Autodesk Fusion 360 part; units mm, degrees
(part 5 of 5)
  line L3475 (115.1928, -67.2452) -> (117.5491, -67.2452)
  line L3476 (117.5491, -67.2452) -> (117.5491, -64.2936)
  line L3477 (117.5491, -64.2936) -> (117.551, -64.2841)
  line L3478 (117.551, -64.2841) -> (117.5645, -64.2705)
  line L3479 (117.5645, -64.2705) -> (117.5741, -64.2686)
  line L3480 (117.5741, -64.2686) -> (131.2663, -64.2686)
  line L3481 (131.2663, -64.2686) -> (131.2758, -64.2705)
  line L3482 (117.5991, -64.3186) -> (117.5991, -67.2702)
  line L3483 (117.5991, -67.2702) -> (117.5972, -67.2798)
  line L3484 (117.5972, -67.2798) -> (117.5836, -67.2933)
  line L3485 (117.5836, -67.2933) -> (117.5741, -67.2952)
  line L3486 (117.5741, -67.2952) -> (115.2178, -67.2952)
  line L3487 (115.2178, -67.2952) -> (115.2178, -70.5194)
  line L3488 (115.2178, -70.5194) -> (117.5741, -70.5194)
  line L3489 (117.5741, -70.5194) -> (117.5836, -70.5213)
  line L3490 (117.5836, -70.5213) -> (117.5972, -70.5348)
  line L3491 (117.5972, -70.5348) -> (117.5991, -70.5444)
  line L3492 (117.5991, -70.5444) -> (117.5991, -72.603)
  line L3493 (117.5991, -72.603) -> (119.9303, -72.603)
  line L3494 (119.9303, -72.603) -> (119.9303, -70.8421)
  line L3495 (119.9303, -70.8421) -> (119.9322, -70.8325)
  line L3496 (119.9322, -70.8325) -> (119.9458, -70.819)
  line L3497 (119.9458, -70.819) -> (119.9553, -70.8171)
  line L3498 (119.9553, -70.8171) -> (121.4436, -70.8171)
  line L3499 (121.4436, -70.8171) -> (121.4532, -70.819)
  line L3500 (121.4532, -70.819) -> (121.4667, -70.8325)
  line L3501 (121.4667, -70.8325) -> (121.4686, -70.8421)
  line L3502 (121.4686, -70.8421) -> (121.4686, -73.7936)
  line L3503 (121.4686, -73.7936) -> (121.7413, -73.7936)
  line L3504 (121.7413, -73.7936) -> (126.1811, -73.7936)
  line L3505 (126.1811, -73.7936) -> (126.1811, -72.628)
  line L3506 (126.1811, -72.628) -> (126.1811, -68.7585)
  line L3507 (126.1811, -68.7585) -> (126.183, -68.7489)
  line L3508 (126.183, -68.7489) -> (126.1965, -68.7354)
  line L3509 (126.1965, -68.7354) -> (126.2061, -68.7335)
  line L3510 (126.2061, -68.7335) -> (128.86, -68.7335)
  line L3511 (128.86, -68.7335) -> (128.86, -67.8655)
  line L3512 (128.86, -67.8655) -> (128.8619, -67.8559)
  line L3513 (128.8619, -67.8559) -> (128.8754, -67.8424)
  line L3514 (128.8754, -67.8424) -> (128.885, -67.8405)
  line L3515 (128.885, -67.8405) -> (131.2413, -67.8405)
  line L3516 (131.2413, -67.8405) -> (131.2413, -64.3186)
  line L3517 (131.2413, -64.3186) -> (117.5991, -64.3186)
  line L3518 (150.3258, -64.2705) -> (150.3394, -64.2841)
  line L3519 (150.3394, -64.2841) -> (150.3413, -64.2936)
  line L3520 (150.3413, -64.2936) -> (150.3413, -67.8655)
  line L3521 (150.3413, -67.8655) -> (150.3394, -67.8751)
  line L3522 (150.3394, -67.8751) -> (150.3258, -67.8886)
  line L3523 (150.3258, -67.8886) -> (150.3163, -67.8905)
  line L3524 (150.3163, -67.8905) -> (147.96, -67.8905)
  line L3525 (147.96, -67.8905) -> (147.96, -68.7585)
  line L3526 (147.96, -68.7585) -> (147.9581, -68.768)
  line L3527 (147.9581, -68.768) -> (147.9446, -68.7816)
  line L3528 (147.9446, -68.7816) -> (147.935, -68.7835)
  line L3529 (147.935, -68.7835) -> (145.2811, -68.7835)
  line L3530 (145.2811, -68.7835) -> (145.2811, -72.628)
  line L3531 (145.2811, -72.628) -> (145.2811, -73.8186)
  line L3532 (145.2811, -73.8186) -> (145.2792, -73.8282)
  line L3533 (145.2792, -73.8282) -> (145.2657, -73.8417)
  line L3534 (145.2657, -73.8417) -> (145.2561, -73.8436)
  line L3535 (145.2561, -73.8436) -> (140.7913, -73.8436)
  line L3536 (140.7913, -73.8436) -> (140.4936, -73.8436)
  line L3537 (140.4936, -73.8436) -> (140.484, -73.8417)
  line L3538 (140.484, -73.8417) -> (140.4705, -73.8282)
  line L3539 (140.4705, -73.8282) -> (140.4686, -73.8186)
  line L3540 (140.4686, -73.8186) -> (140.4686, -70.8671)
  line L3541 (140.4686, -70.8671) -> (139.0303, -70.8671)
  line L3542 (139.0303, -70.8671) -> (139.0303, -72.628)
  line L3543 (139.0303, -72.628) -> (139.0284, -72.6376)
  line L3544 (139.0284, -72.6376) -> (139.0149, -72.6511)
  line L3545 (139.0149, -72.6511) -> (139.0053, -72.653)
  line L3546 (139.0053, -72.653) -> (136.6241, -72.653)
  line L3547 (136.6241, -72.653) -> (136.6145, -72.6511)
  line L3548 (136.6145, -72.6511) -> (136.601, -72.6376)
  line L3549 (136.601, -72.6376) -> (136.5991, -72.628)
  line L3550 (136.5991, -72.628) -> (136.5991, -70.5694)
  line L3551 (136.5991, -70.5694) -> (134.2428, -70.5694)
  line L3552 (134.2428, -70.5694) -> (134.2333, -70.5675)
  line L3553 (134.2333, -70.5675) -> (134.2197, -70.554)
  line L3554 (134.2197, -70.554) -> (134.2178, -70.5444)
  line L3555 (134.2178, -70.5444) -> (134.2178, -67.2702)
  line L3556 (134.2178, -67.2702) -> (134.2197, -67.2606)
  line L3557 (134.2197, -67.2606) -> (134.2333, -67.2471)
  line L3558 (134.2333, -67.2471) -> (134.2428, -67.2452)
  line L3559 (134.2428, -67.2452) -> (136.5991, -67.2452)
  line L3560 (136.5991, -67.2452) -> (136.5991, -64.2936)
  line L3561 (136.5991, -64.2936) -> (136.601, -64.2841)
  line L3562 (136.601, -64.2841) -> (136.6145, -64.2705)
  line L3563 (136.6145, -64.2705) -> (136.6241, -64.2686)
  line L3564 (136.6241, -64.2686) -> (150.3163, -64.2686)
  line L3565 (150.3163, -64.2686) -> (150.3258, -64.2705)
  line L3566 (136.6491, -64.3186) -> (136.6491, -67.2702)
  line L3567 (136.6491, -67.2702) -> (136.6472, -67.2798)
  line L3568 (136.6472, -67.2798) -> (136.6336, -67.2933)
  line L3569 (136.6336, -67.2933) -> (136.6241, -67.2952)
  line L3570 (136.6241, -67.2952) -> (134.2678, -67.2952)
  line L3571 (134.2678, -67.2952) -> (134.2678, -70.5194)
  line L3572 (134.2678, -70.5194) -> (136.6241, -70.5194)
  line L3573 (136.6241, -70.5194) -> (136.6336, -70.5213)
  line L3574 (136.6336, -70.5213) -> (136.6472, -70.5348)
  line L3575 (136.6472, -70.5348) -> (136.6491, -70.5444)
  line L3576 (136.6491, -70.5444) -> (136.6491, -72.603)
  line L3577 (136.6491, -72.603) -> (138.9803, -72.603)
  line L3578 (138.9803, -72.603) -> (138.9803, -70.8421)
  line L3579 (138.9803, -70.8421) -> (138.9822, -70.8325)
  line L3580 (138.9822, -70.8325) -> (138.9958, -70.819)
  line L3581 (138.9958, -70.819) -> (139.0053, -70.8171)
  line L3582 (139.0053, -70.8171) -> (140.4936, -70.8171)
  line L3583 (140.4936, -70.8171) -> (140.5032, -70.819)
  line L3584 (140.5032, -70.819) -> (140.5167, -70.8325)
  line L3585 (140.5167, -70.8325) -> (140.5186, -70.8421)
  line L3586 (140.5186, -70.8421) -> (140.5186, -73.7936)
  line L3587 (140.5186, -73.7936) -> (140.7913, -73.7936)
  line L3588 (140.7913, -73.7936) -> (145.2311, -73.7936)
  line L3589 (145.2311, -73.7936) -> (145.2311, -72.628)
  line L3590 (145.2311, -72.628) -> (145.2311, -68.7585)
  line L3591 (145.2311, -68.7585) -> (145.233, -68.7489)
  line L3592 (145.233, -68.7489) -> (145.2465, -68.7354)
  line L3593 (145.2465, -68.7354) -> (145.2561, -68.7335)
  line L3594 (145.2561, -68.7335) -> (147.91, -68.7335)
  line L3595 (147.91, -68.7335) -> (147.91, -67.8655)
  line L3596 (147.91, -67.8655) -> (147.9119, -67.8559)
  line L3597 (147.9119, -67.8559) -> (147.9254, -67.8424)
  line L3598 (147.9254, -67.8424) -> (147.935, -67.8405)
  line L3599 (147.935, -67.8405) -> (150.2913, -67.8405)
  line L3600 (150.2913, -67.8405) -> (150.2913, -64.3186)
  line L3601 (150.2913, -64.3186) -> (136.6491, -64.3186)
  line L3602 (90.9962, -70.2403) -> (91.2008, -70.2951)
  line L3603 (91.2008, -70.2951) -> (91.3929, -70.3847)
  line L3604 (91.3929, -70.3847) -> (91.5665, -70.5062)
  line L3605 (91.5665, -70.5062) -> (91.7163, -70.6561)
  line L3606 (91.7163, -70.6561) -> (91.8378, -70.8296)
  line L3607 (91.8378, -70.8296) -> (91.9274, -71.0217)
  line L3608 (91.9274, -71.0217) -> (91.9822, -71.2263)
  line L3609 (91.9822, -71.2263) -> (92.0007, -71.4374)
  line L3610 (92.0007, -71.4374) -> (91.9822, -71.6485)
  line L3611 (91.9822, -71.6485) -> (91.9274, -71.8532)
  line L3612 (91.9274, -71.8532) -> (91.8378, -72.0453)
  line L3613 (91.8378, -72.0453) -> (91.7163, -72.2188)
  line L3614 (91.7163, -72.2188) -> (91.5665, -72.3687)
  line L3615 (91.5665, -72.3687) -> (91.3929, -72.4902)
  line L3616 (91.3929, -72.4902) -> (91.2008, -72.5798)
  line L3617 (91.2008, -72.5798) -> (90.9962, -72.6346)
  line L3618 (90.9962, -72.6346) -> (90.7851, -72.6531)
  line L3619 (90.7851, -72.6531) -> (90.574, -72.6346)
  line L3620 (90.574, -72.6346) -> (90.3693, -72.5798)
  line L3621 (90.3693, -72.5798) -> (90.1773, -72.4902)
  line L3622 (90.1773, -72.4902) -> (90.0037, -72.3687)
  line L3623 (90.0037, -72.3687) -> (89.8539, -72.2188)
  line L3624 (89.8539, -72.2188) -> (89.7323, -72.0453)
  line L3625 (89.7323, -72.0453) -> (89.6428, -71.8532)
  line L3626 (89.6428, -71.8532) -> (89.5879, -71.6485)
  line L3627 (89.5879, -71.6485) -> (89.5695, -71.4374)
  line L3628 (89.5695, -71.4374) -> (89.5879, -71.2263)
  line L3629 (89.5879, -71.2263) -> (89.6428, -71.0217)
  line L3630 (89.6428, -71.0217) -> (89.7323, -70.8296)
  line L3631 (89.7323, -70.8296) -> (89.8539, -70.6561)
  line L3632 (89.8539, -70.6561) -> (90.0037, -70.5062)
  line L3633 (90.0037, -70.5062) -> (90.1773, -70.3847)
  line L3634 (90.1773, -70.3847) -> (90.3693, -70.2951)
  line L3635 (90.3693, -70.2951) -> (90.574, -70.2403)
  line L3636 (90.574, -70.2403) -> (90.7851, -70.2218)
  line L3637 (90.7851, -70.2218) -> (90.9962, -70.2403)
  line L3638 (89.6344, -71.6525) -> (89.6935, -71.8603)
  line L3639 (89.6935, -71.8603) -> (89.7898, -72.0537)
  line L3640 (89.7898, -72.0537) -> (89.92, -72.2261)
  line L3641 (89.92, -72.2261) -> (90.0796, -72.3716)
  line L3642 (90.0796, -72.3716) -> (90.2633, -72.4853)
  line L3643 (90.2633, -72.4853) -> (90.4647, -72.5634)
  line L3644 (90.4647, -72.5634) -> (90.6771, -72.6031)
  line L3645 (90.6771, -72.6031) -> (90.8931, -72.6031)
  line L3646 (90.8931, -72.6031) -> (91.1054, -72.5634)
  line L3647 (91.1054, -72.5634) -> (91.3069, -72.4853)
  line L3648 (91.3069, -72.4853) -> (91.4905, -72.3716)
  line L3649 (91.4905, -72.3716) -> (91.6502, -72.2261)
  line L3650 (91.6502, -72.2261) -> (91.7804, -72.0537)
  line L3651 (91.7804, -72.0537) -> (91.8766, -71.8603)
  line L3652 (91.8766, -71.8603) -> (91.9358, -71.6525)
  line L3653 (91.9358, -71.6525) -> (91.9557, -71.4374)
  line L3654 (91.9557, -71.4374) -> (91.9358, -71.2223)
  line L3655 (91.9358, -71.2223) -> (91.8766, -71.0146)
  line L3656 (91.8766, -71.0146) -> (91.7804, -70.8212)
  line L3657 (91.7804, -70.8212) -> (91.6502, -70.6488)
  line L3658 (91.6502, -70.6488) -> (91.4905, -70.5033)
  line L3659 (91.4905, -70.5033) -> (91.3069, -70.3895)
  line L3660 (91.3069, -70.3895) -> (91.1054, -70.3115)
  line L3661 (91.1054, -70.3115) -> (90.8931, -70.2718)
  line L3662 (90.8931, -70.2718) -> (90.6771, -70.2718)
  line L3663 (90.6771, -70.2718) -> (90.4647, -70.3115)
  line L3664 (90.4647, -70.3115) -> (90.2633, -70.3895)
  line L3665 (90.2633, -70.3895) -> (90.0796, -70.5033)
  line L3666 (90.0796, -70.5033) -> (89.92, -70.6488)
  line L3667 (89.92, -70.6488) -> (89.7898, -70.8212)
  line L3668 (89.7898, -70.8212) -> (89.6935, -71.0146)
  line L3669 (89.6935, -71.0146) -> (89.6344, -71.2223)
  line L3670 (89.6344, -71.2223) -> (89.6145, -71.4374)
  line L3671 (89.6145, -71.4374) -> (89.6344, -71.6525)
  line L3672 (110.0462, -70.2403) -> (110.2508, -70.2951)
  line L3673 (110.2508, -70.2951) -> (110.4429, -70.3847)
  line L3674 (110.4429, -70.3847) -> (110.6165, -70.5062)
  line L3675 (110.6165, -70.5062) -> (110.7663, -70.6561)
  line L3676 (110.7663, -70.6561) -> (110.8878, -70.8296)
  line L3677 (110.8878, -70.8296) -> (110.9774, -71.0217)
  line L3678 (110.9774, -71.0217) -> (111.0322, -71.2263)
  line L3679 (111.0322, -71.2263) -> (111.0507, -71.4374)
  line L3680 (111.0507, -71.4374) -> (111.0322, -71.6485)
  line L3681 (111.0322, -71.6485) -> (110.9774, -71.8532)
  line L3682 (110.9774, -71.8532) -> (110.8878, -72.0453)
  line L3683 (110.8878, -72.0453) -> (110.7663, -72.2188)
  line L3684 (110.7663, -72.2188) -> (110.6165, -72.3687)
  line L3685 (110.6165, -72.3687) -> (110.4429, -72.4902)
  line L3686 (110.4429, -72.4902) -> (110.2508, -72.5798)
  line L3687 (110.2508, -72.5798) -> (110.0462, -72.6346)
  line L3688 (110.0462, -72.6346) -> (109.8351, -72.6531)
  line L3689 (109.8351, -72.6531) -> (109.624, -72.6346)
  line L3690 (109.624, -72.6346) -> (109.4193, -72.5798)
  line L3691 (109.4193, -72.5798) -> (109.2273, -72.4902)
  line L3692 (109.2273, -72.4902) -> (109.0537, -72.3687)
  line L3693 (109.0537, -72.3687) -> (108.9038, -72.2188)
  line L3694 (108.9038, -72.2188) -> (108.7823, -72.0453)
  line L3695 (108.7823, -72.0453) -> (108.6928, -71.8532)
  line L3696 (108.6928, -71.8532) -> (108.6379, -71.6485)
  line L3697 (108.6379, -71.6485) -> (108.6194, -71.4374)
  line L3698 (108.6194, -71.4374) -> (108.6379, -71.2263)
  line L3699 (108.6379, -71.2263) -> (108.6928, -71.0217)
  line L3700 (108.6928, -71.0217) -> (108.7823, -70.8296)
  line L3701 (108.7823, -70.8296) -> (108.9038, -70.6561)
  line L3702 (108.9038, -70.6561) -> (109.0537, -70.5062)
  line L3703 (109.0537, -70.5062) -> (109.2273, -70.3847)
  line L3704 (109.2273, -70.3847) -> (109.4193, -70.2951)
  line L3705 (109.4193, -70.2951) -> (109.624, -70.2403)
  line L3706 (109.624, -70.2403) -> (109.8351, -70.2218)
  line L3707 (109.8351, -70.2218) -> (110.0462, -70.2403)
  line L3708 (108.6844, -71.6525) -> (108.7435, -71.8603)
  line L3709 (108.7435, -71.8603) -> (108.8398, -72.0537)
  line L3710 (108.8398, -72.0537) -> (108.97, -72.2261)
  line L3711 (108.97, -72.2261) -> (109.1296, -72.3716)
  line L3712 (109.1296, -72.3716) -> (109.3133, -72.4853)
  line L3713 (109.3133, -72.4853) -> (109.5147, -72.5634)
  line L3714 (109.5147, -72.5634) -> (109.7271, -72.6031)
  line L3715 (109.7271, -72.6031) -> (109.9431, -72.6031)
  line L3716 (109.9431, -72.6031) -> (110.1554, -72.5634)
  line L3717 (110.1554, -72.5634) -> (110.3569, -72.4853)
  line L3718 (110.3569, -72.4853) -> (110.5405, -72.3716)
  line L3719 (110.5405, -72.3716) -> (110.7002, -72.2261)
  line L3720 (110.7002, -72.2261) -> (110.8303, -72.0537)
  line L3721 (110.8303, -72.0537) -> (110.9266, -71.8603)
  line L3722 (110.9266, -71.8603) -> (110.9857, -71.6525)
  line L3723 (110.9857, -71.6525) -> (111.0057, -71.4374)
  line L3724 (111.0057, -71.4374) -> (110.9857, -71.2223)
  line L3725 (110.9857, -71.2223) -> (110.9266, -71.0146)
  line L3726 (110.9266, -71.0146) -> (110.8303, -70.8212)
  line L3727 (110.8303, -70.8212) -> (110.7002, -70.6488)
  line L3728 (110.7002, -70.6488) -> (110.5405, -70.5033)
  line L3729 (110.5405, -70.5033) -> (110.3569, -70.3895)
  line L3730 (110.3569, -70.3895) -> (110.1554, -70.3115)
  line L3731 (110.1554, -70.3115) -> (109.9431, -70.2718)
  line L3732 (109.9431, -70.2718) -> (109.7271, -70.2718)
  line L3733 (109.7271, -70.2718) -> (109.5147, -70.3115)
  line L3734 (109.5147, -70.3115) -> (109.3133, -70.3895)
  line L3735 (109.3133, -70.3895) -> (109.1296, -70.5033)
  line L3736 (109.1296, -70.5033) -> (108.97, -70.6488)
  line L3737 (108.97, -70.6488) -> (108.8398, -70.8212)
  line L3738 (108.8398, -70.8212) -> (108.7435, -71.0146)
  line L3739 (108.7435, -71.0146) -> (108.6844, -71.2223)
  line L3740 (108.6844, -71.2223) -> (108.6644, -71.4374)
  line L3741 (108.6644, -71.4374) -> (108.6844, -71.6525)
  line L3742 (129.0961, -70.2402) -> (129.3008, -70.2951)
  line L3743 (129.3008, -70.2951) -> (129.4928, -70.3846)
  line L3744 (129.4928, -70.3846) -> (129.6664, -70.5062)
  line L3745 (129.6664, -70.5062) -> (129.8162, -70.656)
  line L3746 (129.8162, -70.656) -> (129.9378, -70.8296)
  line L3747 (129.9378, -70.8296) -> (130.0273, -71.0216)
  line L3748 (130.0273, -71.0216) -> (130.0822, -71.2263)
  line L3749 (130.0822, -71.2263) -> (130.1006, -71.4374)
  line L3750 (130.1006, -71.4374) -> (130.0822, -71.6485)
  line L3751 (130.0822, -71.6485) -> (130.0273, -71.8531)
  line L3752 (130.0273, -71.8531) -> (129.9378, -72.0452)
  line L3753 (129.9378, -72.0452) -> (129.8162, -72.2188)
  line L3754 (129.8162, -72.2188) -> (129.6664, -72.3686)
  line L3755 (129.6664, -72.3686) -> (129.4928, -72.4901)
  line L3756 (129.4928, -72.4901) -> (129.3008, -72.5797)
  line L3757 (129.3008, -72.5797) -> (129.0961, -72.6345)
  line L3758 (129.0961, -72.6345) -> (128.885, -72.653)
  line L3759 (128.885, -72.653) -> (128.6739, -72.6345)
  line L3760 (128.6739, -72.6345) -> (128.4692, -72.5797)
  line L3761 (128.4692, -72.5797) -> (128.2772, -72.4901)
  line L3762 (128.2772, -72.4901) -> (128.1036, -72.3686)
  line L3763 (128.1036, -72.3686) -> (127.9538, -72.2188)
  line L3764 (127.9538, -72.2188) -> (127.8322, -72.0452)
  line L3765 (127.8322, -72.0452) -> (127.7427, -71.8531)
  line L3766 (127.7427, -71.8531) -> (127.6879, -71.6485)
  line L3767 (127.6879, -71.6485) -> (127.6694, -71.4374)
  line L3768 (127.6694, -71.4374) -> (127.6879, -71.2263)
  line L3769 (127.6879, -71.2263) -> (127.7427, -71.0216)
  line L3770 (127.7427, -71.0216) -> (127.8322, -70.8296)
  line L3771 (127.8322, -70.8296) -> (127.9538, -70.656)
  line L3772 (127.9538, -70.656) -> (128.1036, -70.5062)
  line L3773 (128.1036, -70.5062) -> (128.2772, -70.3846)
  line L3774 (128.2772, -70.3846) -> (128.4692, -70.2951)
  line L3775 (128.4692, -70.2951) -> (128.6739, -70.2402)
  line L3776 (128.6739, -70.2402) -> (128.885, -70.2218)
  line L3777 (128.885, -70.2218) -> (129.0961, -70.2402)
  line L3778 (127.7343, -71.6525) -> (127.7934, -71.8603)
  line L3779 (127.7934, -71.8603) -> (127.8897, -72.0536)
  line L3780 (127.8897, -72.0536) -> (128.0199, -72.226)
  line L3781 (128.0199, -72.226) -> (128.1796, -72.3715)
  line L3782 (128.1796, -72.3715) -> (128.3632, -72.4853)
  line L3783 (128.3632, -72.4853) -> (128.5647, -72.5633)
  line L3784 (128.5647, -72.5633) -> (128.777, -72.603)
  line L3785 (128.777, -72.603) -> (128.993, -72.603)
  line L3786 (128.993, -72.603) -> (129.2054, -72.5633)
  line L3787 (129.2054, -72.5633) -> (129.4068, -72.4853)
  line L3788 (129.4068, -72.4853) -> (129.5905, -72.3715)
  line L3789 (129.5905, -72.3715) -> (129.7501, -72.226)
  line L3790 (129.7501, -72.226) -> (129.8803, -72.0536)
  line L3791 (129.8803, -72.0536) -> (129.9766, -71.8603)
  line L3792 (129.9766, -71.8603) -> (130.0357, -71.6525)
  line L3793 (130.0357, -71.6525) -> (130.0556, -71.4374)
  line L3794 (130.0556, -71.4374) -> (130.0357, -71.2223)
  line L3795 (130.0357, -71.2223) -> (129.9766, -71.0145)
  line L3796 (129.9766, -71.0145) -> (129.8803, -70.8211)
  line L3797 (129.8803, -70.8211) -> (129.7501, -70.6487)
  line L3798 (129.7501, -70.6487) -> (129.5905, -70.5032)
  line L3799 (129.5905, -70.5032) -> (129.4068, -70.3895)
  line L3800 (129.4068, -70.3895) -> (129.2054, -70.3114)
  line L3801 (129.2054, -70.3114) -> (128.993, -70.2718)
  line L3802 (128.993, -70.2718) -> (128.777, -70.2718)
  line L3803 (128.777, -70.2718) -> (128.5647, -70.3114)
  line L3804 (128.5647, -70.3114) -> (128.3632, -70.3895)
  line L3805 (128.3632, -70.3895) -> (128.1796, -70.5032)
  line L3806 (128.1796, -70.5032) -> (128.0199, -70.6487)
  line L3807 (128.0199, -70.6487) -> (127.8897, -70.8211)
  line L3808 (127.8897, -70.8211) -> (127.7934, -71.0145)
  line L3809 (127.7934, -71.0145) -> (127.7343, -71.2223)
  line L3810 (127.7343, -71.2223) -> (127.7144, -71.4374)
  line L3811 (127.7144, -71.4374) -> (127.7343, -71.6525)
  line L3812 (148.1461, -70.2402) -> (148.3508, -70.2951)
  line L3813 (148.3508, -70.2951) -> (148.5428, -70.3846)
  line L3814 (148.5428, -70.3846) -> (148.7164, -70.5062)
  line L3815 (148.7164, -70.5062) -> (148.8662, -70.656)
  line L3816 (148.8662, -70.656) -> (148.9878, -70.8296)
  line L3817 (148.9878, -70.8296) -> (149.0773, -71.0216)
  line L3818 (149.0773, -71.0216) -> (149.1322, -71.2263)
  line L3819 (149.1322, -71.2263) -> (149.1506, -71.4374)
  line L3820 (149.1506, -71.4374) -> (149.1322, -71.6485)
  line L3821 (149.1322, -71.6485) -> (149.0773, -71.8531)
  line L3822 (149.0773, -71.8531) -> (148.9878, -72.0452)
  line L3823 (148.9878, -72.0452) -> (148.8662, -72.2188)
  line L3824 (148.8662, -72.2188) -> (148.7164, -72.3686)
  line L3825 (148.7164, -72.3686) -> (148.5428, -72.4901)
  line L3826 (148.5428, -72.4901) -> (148.3508, -72.5797)
  line L3827 (148.3508, -72.5797) -> (148.1461, -72.6345)
  line L3828 (148.1461, -72.6345) -> (147.935, -72.653)
  line L3829 (147.935, -72.653) -> (147.7239, -72.6345)
  line L3830 (147.7239, -72.6345) -> (147.5192, -72.5797)
  line L3831 (147.5192, -72.5797) -> (147.3272, -72.4901)
  line L3832 (147.3272, -72.4901) -> (147.1536, -72.3686)
  line L3833 (147.1536, -72.3686) -> (147.0038, -72.2188)
  line L3834 (147.0038, -72.2188) -> (146.8822, -72.0452)
  line L3835 (146.8822, -72.0452) -> (146.7927, -71.8531)
  line L3836 (146.7927, -71.8531) -> (146.7379, -71.6485)
  line L3837 (146.7379, -71.6485) -> (146.7194, -71.4374)
  line L3838 (146.7194, -71.4374) -> (146.7379, -71.2263)
  line L3839 (146.7379, -71.2263) -> (146.7927, -71.0216)
  line L3840 (146.7927, -71.0216) -> (146.8822, -70.8296)
  line L3841 (146.8822, -70.8296) -> (147.0038, -70.656)
  line L3842 (147.0038, -70.656) -> (147.1536, -70.5062)
  line L3843 (147.1536, -70.5062) -> (147.3272, -70.3846)
  line L3844 (147.3272, -70.3846) -> (147.5192, -70.2951)
  line L3845 (147.5192, -70.2951) -> (147.7239, -70.2402)
  line L3846 (147.7239, -70.2402) -> (147.935, -70.2218)
  line L3847 (147.935, -70.2218) -> (148.1461, -70.2402)
  line L3848 (146.7843, -71.6525) -> (146.8434, -71.8603)
  line L3849 (146.8434, -71.8603) -> (146.9397, -72.0536)
  line L3850 (146.9397, -72.0536) -> (147.0699, -72.226)
  line L3851 (147.0699, -72.226) -> (147.2296, -72.3715)
  line L3852 (147.2296, -72.3715) -> (147.4132, -72.4853)
  line L3853 (147.4132, -72.4853) -> (147.6147, -72.5633)
  line L3854 (147.6147, -72.5633) -> (147.827, -72.603)
  line L3855 (147.827, -72.603) -> (148.043, -72.603)
  line L3856 (148.043, -72.603) -> (148.2554, -72.5633)
  line L3857 (148.2554, -72.5633) -> (148.4568, -72.4853)
  line L3858 (148.4568, -72.4853) -> (148.6405, -72.3715)
  line L3859 (148.6405, -72.3715) -> (148.8001, -72.226)
  line L3860 (148.8001, -72.226) -> (148.9303, -72.0536)
  line L3861 (148.9303, -72.0536) -> (149.0266, -71.8603)
  line L3862 (149.0266, -71.8603) -> (149.0857, -71.6525)
  line L3863 (149.0857, -71.6525) -> (149.1056, -71.4374)
  line L3864 (149.1056, -71.4374) -> (149.0857, -71.2223)
  line L3865 (149.0857, -71.2223) -> (149.0266, -71.0145)
  line L3866 (149.0266, -71.0145) -> (148.9303, -70.8211)
  line L3867 (148.9303, -70.8211) -> (148.8001, -70.6487)
  line L3868 (148.8001, -70.6487) -> (148.6405, -70.5032)
  line L3869 (148.6405, -70.5032) -> (148.4568, -70.3895)
  line L3870 (148.4568, -70.3895) -> (148.2554, -70.3114)
  line L3871 (148.2554, -70.3114) -> (148.043, -70.2718)
  line L3872 (148.043, -70.2718) -> (147.827, -70.2718)
  line L3873 (147.827, -70.2718) -> (147.6147, -70.3114)
  line L3874 (147.6147, -70.3114) -> (147.4132, -70.3895)
  line L3875 (147.4132, -70.3895) -> (147.2296, -70.5032)
  line L3876 (147.2296, -70.5032) -> (147.0699, -70.6487)
  line L3877 (147.0699, -70.6487) -> (146.9397, -70.8211)
  line L3878 (146.9397, -70.8211) -> (146.8434, -71.0145)
  line L3879 (146.8434, -71.0145) -> (146.7843, -71.2223)
  line L3880 (146.7843, -71.2223) -> (146.7644, -71.4374)
  line L3881 (146.7644, -71.4374) -> (146.7843, -71.6525)
  line L3882 (150.4, -61.8625) -> (150.6676, -61.88)
  line L3883 (150.6676, -61.88) -> (150.9306, -61.9324)
  line L3884 (150.9306, -61.9324) -> (151.1845, -62.0185)
  line L3885 (151.1845, -62.0185) -> (151.425, -62.1371)
  line L3886 (151.425, -62.1371) -> (151.648, -62.2861)
  line L3887 (151.648, -62.2861) -> (151.8496, -62.4629)
  line L3888 (151.8496, -62.4629) -> (152.0264, -62.6645)
  line L3889 (152.0264, -62.6645) -> (152.1754, -62.8875)
  line L3890 (152.1754, -62.8875) -> (152.294, -63.128)
  line L3891 (152.294, -63.128) -> (152.3801, -63.3819)
  line L3892 (152.3801, -63.3819) -> (152.4325, -63.6449)
  line L3893 (152.4325, -63.6449) -> (152.45, -63.9125)
  line L3894 (152.45, -63.9125) -> (152.4405, -63.9419)
  line L3895 (152.4405, -63.9419) -> (152.425, -63.9531)
  line L3896 (152.425, -63.9531) -> (152.4249, -123.5272)
  line L3897 (152.4249, -123.5272) -> (152.423, -123.5368)
  line L3898 (152.423, -123.5368) -> (152.4094, -123.5503)
  line L3899 (152.4094, -123.5503) -> (152.3999, -123.5522)
  line L3900 (152.3999, -123.5522) -> (132.1843, -123.5522)
  line L3901 (132.1843, -123.5522) -> (132.1843, -128.86)
  line L3902 (132.1843, -128.86) -> (143.7681, -128.86)
  line L3903 (143.7681, -128.86) -> (143.7777, -128.862)
  line L3904 (143.7777, -128.862) -> (143.7912, -128.8755)
  line L3905 (143.7912, -128.8755) -> (143.7931, -128.885)
  line L3906 (143.7931, -128.885) -> (143.7931, -131.8616)
  line L3907 (143.7931, -131.8616) -> (143.7912, -131.8711)
  line L3908 (143.7912, -131.8711) -> (143.7912, -131.8711)
  line L3909 (143.7912, -131.8711) -> (143.7777, -131.8847)
  line L3910 (143.7777, -131.8847) -> (143.7681, -131.8866)
  line L3911 (143.7681, -131.8866) -> (141.7095, -131.8866)
  line L3912 (141.7095, -131.8866) -> (141.7095, -134.2178)
  line L3913 (141.7095, -134.2178) -> (143.4704, -134.2178)
  line L3914 (143.4704, -134.2178) -> (143.48, -134.2197)
  line L3915 (143.48, -134.2197) -> (143.4935, -134.2333)
  line L3916 (143.4935, -134.2333) -> (143.4954, -134.2428)
  line L3917 (143.4954, -134.2428) -> (143.4954, -135.7311)
  line L3918 (143.4954, -135.7311) -> (143.4935, -135.7407)
  line L3919 (143.4935, -135.7407) -> (143.48, -135.7542)
  line L3920 (143.48, -135.7542) -> (143.4704, -135.7561)
  line L3921 (143.4704, -135.7561) -> (140.5189, -135.7561)
  line L3922 (140.5189, -135.7561) -> (140.5189, -136.0288)
  line L3923 (140.5189, -136.0288) -> (140.5189, -140.4686)
  line L3924 (140.5189, -140.4686) -> (141.6845, -140.4686)
  line L3925 (141.6845, -140.4686) -> (145.554, -140.4686)
  line L3926 (145.554, -140.4686) -> (145.5636, -140.4705)
  line L3927 (145.5636, -140.4705) -> (145.5771, -140.484)
  line L3928 (145.5771, -140.484) -> (145.579, -140.4936)
  line L3929 (145.579, -140.4936) -> (145.579, -143.1475)
  line L3930 (145.579, -143.1475) -> (146.447, -143.1475)
  line L3931 (146.447, -143.1475) -> (146.4566, -143.1494)
  line L3932 (146.4566, -143.1494) -> (146.4701, -143.1629)
  line L3933 (146.4701, -143.1629) -> (146.472, -143.1725)
  line L3934 (146.472, -143.1725) -> (146.472, -145.5288)
  line L3935 (146.472, -145.5288) -> (149.9939, -145.5288)
  line L3936 (149.9939, -145.5288) -> (149.9939, -131.8866)
  line L3937 (149.9939, -131.8866) -> (147.0423, -131.8866)
  line L3938 (147.0423, -131.8866) -> (147.0327, -131.8847)
  line L3939 (147.0327, -131.8847) -> (147.0327, -131.8847)
  line L3940 (147.0327, -131.8847) -> (147.0327, -131.8847)
  line L3941 (147.0327, -131.8847) -> (147.0327, -131.8847)
  line L3942 (147.0327, -131.8847) -> (147.026, -131.8779)
  line L3943 (147.026, -131.8779) -> (147.0192, -131.8711)
  line L3944 (147.0192, -131.8711) -> (147.0192, -131.8711)
  line L3945 (147.0192, -131.8711) -> (147.0192, -131.8711)
  line L3946 (147.0192, -131.8711) -> (147.0173, -131.8616)
  line L3947 (147.0173, -131.8616) -> (147.0171, -128.8851)
  line L3948 (147.0171, -128.8851) -> (147.019, -128.8755)
  line L3949 (147.019, -128.8755) -> (147.019, -128.8755)
  line L3950 (147.019, -128.8755) -> (147.0257, -128.8687)
  line L3951 (147.0257, -128.8687) -> (147.0325, -128.862)
  line L3952 (147.0325, -128.862) -> (147.0325, -128.862)
  line L3953 (147.0325, -128.862) -> (147.0325, -128.862)
  line L3954 (147.0325, -128.862) -> (147.0421, -128.86)
  line L3955 (147.0421, -128.86) -> (152.3999, -128.86)
  line L3956 (152.3999, -128.86) -> (152.4094, -128.862)
  line L3957 (152.4094, -128.862) -> (152.423, -128.8755)
  line L3958 (152.423, -128.8755) -> (152.4249, -128.885)
  line L3959 (152.4249, -128.885) -> (152.4249, -147.3397)
  line L3960 (152.4249, -147.3397) -> (152.423, -147.3493)
  line L3961 (152.423, -147.3493) -> (152.4094, -147.3628)
  line L3962 (152.4094, -147.3628) -> (152.3999, -147.3647)
  line L3963 (152.3999, -147.3647) -> (132.1843, -147.3647)
  line L3964 (132.1843, -147.3647) -> (132.1843, -152.6725)
  line L3965 (132.1843, -152.6725) -> (152.3595, -152.6725)
  line L3966 (152.3595, -152.6725) -> (152.3807, -152.6513)
  line L3967 (152.3807, -152.6513) -> (152.419, -152.6513)
  line L3968 (152.419, -152.6513) -> (152.4461, -152.6784)
  line L3969 (152.4461, -152.6784) -> (152.4499, -152.6975)
  line L3970 (152.4499, -152.6975) -> (152.45, -155.1625)
  line L3971 (152.45, -155.1625) -> (152.45, -155.1625)
  line L3972 (152.45, -155.1625) -> (152.45, -155.1625)
  line L3973 (152.45, -155.1625) -> (152.4325, -155.4301)
  line L3974 (152.4325, -155.4301) -> (152.3801, -155.6931)
  line L3975 (152.3801, -155.6931) -> (152.294, -155.947)
  line L3976 (152.294, -155.947) -> (152.1754, -156.1875)
  line L3977 (152.1754, -156.1875) -> (152.0264, -156.4105)
  line L3978 (152.0264, -156.4105) -> (151.8496, -156.6121)
  line L3979 (151.8496, -156.6121) -> (151.648, -156.7889)
  line L3980 (151.648, -156.7889) -> (151.425, -156.9379)
  line L3981 (151.425, -156.9379) -> (151.1845, -157.0565)
  line L3982 (151.1845, -157.0565) -> (150.9306, -157.1426)
  line L3983 (150.9306, -157.1426) -> (150.6676, -157.195)
  line L3984 (150.6676, -157.195) -> (150.4, -157.2125)
  line L3985 (150.4, -157.2125) -> (54.3875, -157.2125)
  line L3986 (54.3875, -157.2125) -> (54.1199, -157.195)
  line L3987 (54.1199, -157.195) -> (53.8569, -157.1426)
  line L3988 (53.8569, -157.1426) -> (53.603, -157.0565)
  line L3989 (53.603, -157.0565) -> (53.3625, -156.9379)
  line L3990 (53.3625, -156.9379) -> (53.1395, -156.7889)
  line L3991 (53.1395, -156.7889) -> (52.9379, -156.6121)
  line L3992 (52.9379, -156.6121) -> (52.7611, -156.4105)
  line L3993 (52.7611, -156.4105) -> (52.6121, -156.1875)
  line L3994 (52.6121, -156.1875) -> (52.4935, -155.947)
  line L3995 (52.4935, -155.947) -> (52.4074, -155.6931)
  line L3996 (52.4074, -155.6931) -> (52.355, -155.4301)
  line L3997 (52.355, -155.4301) -> (52.3375, -155.1625)
  line L3998 (52.3375, -155.1625) -> (52.3375, -86.3202)
  line L3999 (52.3375, -86.3202) -> (52.3413, -86.3011)
  line L4000 (52.3413, -86.3011) -> (52.3683, -86.274)
  line L4001 (52.3683, -86.274) -> (52.4066, -86.274)
  line L4002 (52.4066, -86.274) -> (52.4278, -86.2952)
  line L4003 (52.4278, -86.2952) -> (55.364, -86.2952)
  line L4004 (55.364, -86.2952) -> (74.6867, -86.2952)
  line L4005 (74.6867, -86.2952) -> (74.6867, -61.9528)
  line L4006 (74.6867, -61.9528) -> (74.6655, -61.9316)
  line L4007 (74.6655, -61.9316) -> (74.6655, -61.8933)
  line L4008 (74.6655, -61.8933) -> (74.6925, -61.8663)
  line L4009 (74.6925, -61.8663) -> (74.7117, -61.8624)
  line L4010 (74.7117, -61.8624) -> (150.4, -61.8625)
  line L4011 (74.7367, -86.3202) -> (74.7348, -86.3298)
  line L4012 (74.7348, -86.3298) -> (74.7212, -86.3433)
  line L4013 (74.7212, -86.3433) -> (74.7117, -86.3452)
  line L4014 (74.7117, -86.3452) -> (55.364, -86.3452)
  line L4015 (55.364, -86.3452) -> (52.4375, -86.3452)
  line L4016 (52.4375, -86.3452) -> (52.4375, -155.1625)
  line L4017 (52.4375, -155.1625) -> (52.4375, -155.2903)
  line L4018 (52.4375, -155.2903) -> (52.4709, -155.5437)
  line L4019 (52.4709, -155.5437) -> (52.537, -155.7907)
  line L4020 (52.537, -155.7907) -> (52.6348, -156.0268)
  line L4021 (52.6348, -156.0268) -> (52.7627, -156.2482)
  line L4022 (52.7627, -156.2482) -> (52.9183, -156.451)
  line L4023 (52.9183, -156.451) -> (53.099, -156.6317)
  line L4024 (53.099, -156.6317) -> (53.3018, -156.7873)
  line L4025 (53.3018, -156.7873) -> (53.5232, -156.9152)
  line L4026 (53.5232, -156.9152) -> (53.7593, -157.013)
  line L4027 (53.7593, -157.013) -> (54.0063, -157.0791)
  line L4028 (54.0063, -157.0791) -> (54.2597, -157.1125)
  line L4029 (54.2597, -157.1125) -> (54.3875, -157.1125)
  line L4030 (54.3875, -157.1125) -> (150.4, -157.1125)
  line L4031 (150.4, -157.1125) -> (150.5278, -157.1125)
  line L4032 (150.5278, -157.1125) -> (150.7812, -157.0791)
  line L4033 (150.7812, -157.0791) -> (151.0282, -157.013)
  line L4034 (151.0282, -157.013) -> (151.2643, -156.9152)
  line L4035 (151.2643, -156.9152) -> (151.4857, -156.7873)
  line L4036 (151.4857, -156.7873) -> (151.6885, -156.6317)
  line L4037 (151.6885, -156.6317) -> (151.8692, -156.451)
  line L4038 (151.8692, -156.451) -> (152.0248, -156.2482)
  line L4039 (152.0248, -156.2482) -> (152.1527, -156.0268)
  line L4040 (152.1527, -156.0268) -> (152.2505, -155.7907)
  line L4041 (152.2505, -155.7907) -> (152.3166, -155.5437)
  line L4042 (152.3166, -155.5437) -> (152.35, -155.2903)
  line L4043 (152.35, -155.2903) -> (152.35, -155.1625)
  line L4044 (152.35, -155.1625) -> (152.3499, -152.7225)
  line L4045 (152.3499, -152.7225) -> (132.1593, -152.7225)
  line L4046 (132.1593, -152.7225) -> (132.1497, -152.7206)
  line L4047 (132.1497, -152.7206) -> (132.1362, -152.7071)
  line L4048 (132.1362, -152.7071) -> (132.1343, -152.6975)
  line L4049 (132.1343, -152.6975) -> (132.1343, -147.3397)
  line L4050 (132.1343, -147.3397) -> (132.1362, -147.3302)
  line L4051 (132.1362, -147.3302) -> (132.1497, -147.3166)
  line L4052 (132.1497, -147.3166) -> (132.1593, -147.3147)
  line L4053 (132.1593, -147.3147) -> (152.3749, -147.3147)
  line L4054 (152.3749, -147.3147) -> (152.3749, -128.91)
  line L4055 (152.3749, -128.91) -> (147.0671, -128.91)
  line L4056 (147.0671, -128.91) -> (147.0673, -131.8366)
  line L4057 (147.0673, -131.8366) -> (150.0189, -131.8366)
  line L4058 (150.0189, -131.8366) -> (150.0284, -131.8385)
  line L4059 (150.0284, -131.8385) -> (150.042, -131.852)
  line L4060 (150.042, -131.852) -> (150.0439, -131.8616)
  line L4061 (150.0439, -131.8616) -> (150.0439, -145.5538)
  line L4062 (150.0439, -145.5538) -> (150.042, -145.5633)
  line L4063 (150.042, -145.5633) -> (150.0284, -145.5769)
  line L4064 (150.0284, -145.5769) -> (150.0189, -145.5788)
  line L4065 (150.0189, -145.5788) -> (146.447, -145.5788)
  line L4066 (146.447, -145.5788) -> (146.4374, -145.5769)
  line L4067 (146.4374, -145.5769) -> (146.4239, -145.5633)
  line L4068 (146.4239, -145.5633) -> (146.422, -145.5538)
  line L4069 (146.422, -145.5538) -> (146.422, -143.1975)
  line L4070 (146.422, -143.1975) -> (145.554, -143.1975)
  line L4071 (145.554, -143.1975) -> (145.5445, -143.1956)
  line L4072 (145.5445, -143.1956) -> (145.5309, -143.1821)
  line L4073 (145.5309, -143.1821) -> (145.529, -143.1725)
  line L4074 (145.529, -143.1725) -> (145.529, -140.5186)
  line L4075 (145.529, -140.5186) -> (141.6845, -140.5186)
  line L4076 (141.6845, -140.5186) -> (140.4939, -140.5186)
  line L4077 (140.4939, -140.5186) -> (140.4843, -140.5167)
  line L4078 (140.4843, -140.5167) -> (140.4708, -140.5032)
  line L4079 (140.4708, -140.5032) -> (140.4689, -140.4936)
  line L4080 (140.4689, -140.4936) -> (140.4689, -136.0288)
  line L4081 (140.4689, -136.0288) -> (140.4689, -135.7311)
  line L4082 (140.4689, -135.7311) -> (140.4708, -135.7215)
  line L4083 (140.4708, -135.7215) -> (140.4843, -135.708)
  line L4084 (140.4843, -135.708) -> (140.4939, -135.7061)
  line L4085 (140.4939, -135.7061) -> (143.4454, -135.7061)
  line L4086 (143.4454, -135.7061) -> (143.4454, -134.2678)
  line L4087 (143.4454, -134.2678) -> (141.6845, -134.2678)
  line L4088 (141.6845, -134.2678) -> (141.6749, -134.2659)
  line L4089 (141.6749, -134.2659) -> (141.6614, -134.2524)
  line L4090 (141.6614, -134.2524) -> (141.6595, -134.2428)
  line L4091 (141.6595, -134.2428) -> (141.6595, -131.8616)
  line L4092 (141.6595, -131.8616) -> (141.6614, -131.852)
  line L4093 (141.6614, -131.852) -> (141.6749, -131.8385)
  line L4094 (141.6749, -131.8385) -> (141.6845, -131.8366)
  line L4095 (141.6845, -131.8366) -> (143.7431, -131.8366)
  line L4096 (143.7431, -131.8366) -> (143.7431, -128.91)
  line L4097 (143.7431, -128.91) -> (132.1593, -128.91)
  line L4098 (132.1593, -128.91) -> (132.1497, -128.9081)
  line L4099 (132.1497, -128.9081) -> (132.1362, -128.8946)
  line L4100 (132.1362, -128.8946) -> (132.1343, -128.885)
  line L4101 (132.1343, -128.885) -> (132.1343, -123.5272)
  line L4102 (132.1343, -123.5272) -> (132.1362, -123.5177)
  line L4103 (132.1362, -123.5177) -> (132.1497, -123.5041)
  line L4104 (132.1497, -123.5041) -> (132.1593, -123.5022)
  line L4105 (132.1593, -123.5022) -> (152.3749, -123.5022)
  line L4106 (152.3749, -123.5022) -> (152.375, -63.9531)
  line L4107 (152.375, -63.9531) -> (152.3595, -63.9419)
  line L4108 (152.3595, -63.9419) -> (152.35, -63.9125)
  line L4109 (152.35, -63.9125) -> (152.35, -63.7847)
  line L4110 (152.35, -63.7847) -> (152.3166, -63.5313)
  line L4111 (152.3166, -63.5313) -> (152.2505, -63.2843)
  line L4112 (152.2505, -63.2843) -> (152.1527, -63.0482)
  line L4113 (152.1527, -63.0482) -> (152.0248, -62.8268)
  line L4114 (152.0248, -62.8268) -> (151.8692, -62.624)
  line L4115 (151.8692, -62.624) -> (151.6885, -62.4433)
  line L4116 (151.6885, -62.4433) -> (151.4857, -62.2877)
  line L4117 (151.4857, -62.2877) -> (151.2643, -62.1598)
  line L4118 (151.2643, -62.1598) -> (151.0282, -62.062)
  line L4119 (151.0282, -62.062) -> (150.7812, -61.9959)
  line L4120 (150.7812, -61.9959) -> (150.5278, -61.9625)
  line L4121 (150.5278, -61.9625) -> (150.4, -61.9625)
  line L4122 (150.4, -61.9625) -> (74.7367, -61.9624)
  line L4123 (74.7367, -61.9624) -> (74.7367, -86.3202)
extrude "押し出し1" add sketch "スケッチ1" along normal blind 2 contours L4011 L4012 L4013 L4014 L4015 L4016 L4017 L4018 L4019 L4020 L4021 L4022 L4023 L4024 L4025 L4026 L4027 L4028 L4029 L4030 L4031 L4032 L4033 L4034 L4035 L4036 L4037 L4038 L4039 L4040 L4041 L4042 L4043 L4044 L4045 L4046 L4047 L4048 L4049 L4050 L4051 L4052 L4053 L4054 L4055 L4056 L4057 L4058 L4059 L4060 L4061 L4062 L4063 L4064 L4065 L4066 L4067 L4068 L4069 L4070 L4071 L4072 L4073 L4074 L4075 L4076 L4077 L4078 L4079 L4080 L4081 L4082 L4083 L4084 L4085 L4086 L4087 L4088 L4089 L4090 L4091 L4092 L4093 L4094 L4095 L4096 L4097 L4098 L4099 L4100 L4101 L4102 L4103 L4104 L4105 L4106 L4107 L4108 L4109 L4110 L4111 L4112 L4113 L4114 L4115 L4116 L4117 L4118 L4119 L4120 L4121 L4122 L4123
